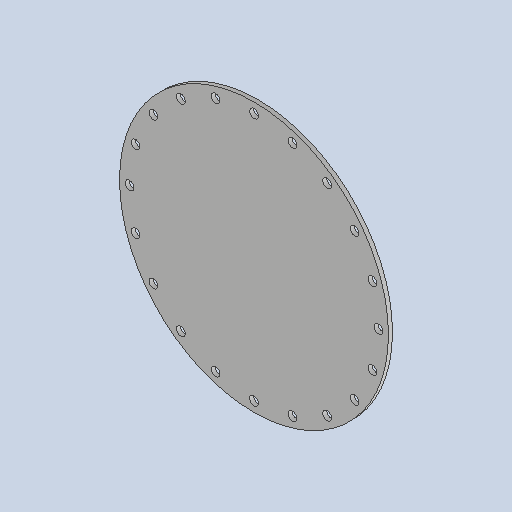
# Autodesk Inventor part: SLM 1621 charging hatch D940_1200
Saved by Autodesk Inventor 2026.2 (Build 302298000, 298)
## iProperties
Created: 2025-02-12
Part Number: SLM 1621 charging hatch D940_1200
Material: Generic
Document SubType Name: Sheet Metal
Designer: admin
Density: 1 g/cm^3
Flat Pattern Width: 67 cm
Flat Pattern Length: 67 cm
Flat Pattern Area: 4489 cm^2
Sheet Metal Rule: Default_mm
Sheet Metal Width: 670,000 mm
Sheet Metal Length: 670,000 mm
Sheet Metal Area: 448900,000 mm^2
Appearance: Default
Author: pokla
Autodesk Inventor part; units mm, degrees
ref_plane "YZ Plane" through (0, 0, 0) normal (1, 0, 0) x (0, 1, 0)
ref_plane "XZ Plane" through (0, 0, 0) normal (0, 1, 0) x (-1, 0, 0)
ref_plane "XY Plane" through (0, 0, 0) normal (0, 0, 1) x (1, 0, 0)
sketch "Sketch1" plane through (0, 0, 0) normal (0, 1, 0) x (-1, 0, 0)
  circle A0 centre (0, 0) radius 335
  dimension "d0" = 670
  constraints: 1 centre point, 1 coincident
  measures "d0" diameter of A0
extrude "Extrusion1" add sketch "Sketch1" along normal blind 10
sketch "Sketch2" plane through (0, 10, 0) normal (0, 1, 0) x (1, 0, 0)
  circle A0 centre (-310, 0) radius 11
  circle A1 centre (0, 0) radius 310 construction
  dimension "d4" = 620
  dimension "d3" = 22
  constraints: 2 horizontal alignment, 1 centre point, 1 coincident, 2 other
  measures "d3" diameter of A0
extrude "Cut1" cut sketch "Sketch2" against normal blind 10
pattern_circular "Circular Pattern1" count 20 over 360 about axis through (0, 0, 0) along (0, 1, 0) of "Cut1"
equation "\"d1\" = Thickness"
equation "\"d6\" = Thickness"
equation "\"BendReliefDepth\" = 0.5 * Thickness"
equation "\"Thickness\" = 10"
body "Solid1"
